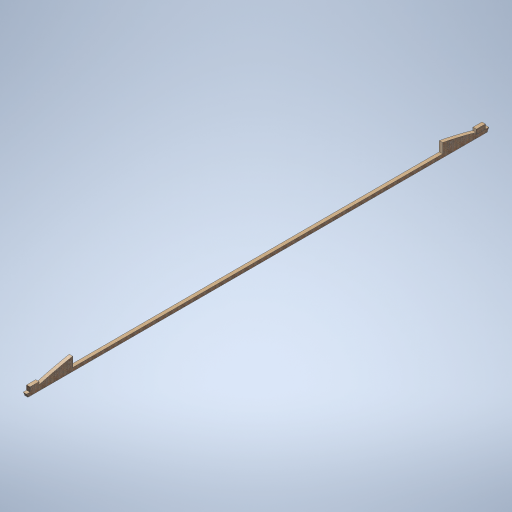
# Autodesk Inventor part: main_crossbeam
Saved by Autodesk Inventor 2024.2 (Build 282272000, 272)
## iProperties
Created: 2024-05-18
Part Number: main_crossbeam
Material: Wood Shake
Document SubType Name: Modeling
Designer: LOSTER_1
Density: 0.4 g/cm^3
Appearance: Shake - Handsplit
Author: LOSTER_1
Autodesk Inventor part; units mm, degrees
ref_plane "YZ Plane" through (0, 0, 0) normal (1, 0, 0) x (0, 1, 0)
ref_plane "XZ Plane" through (0, 0, 0) normal (0, 1, 0) x (-1, 0, 0)
ref_plane "XY Plane" through (0, 0, 0) normal (0, 0, 1) x (1, 0, 0)
sketch "Sketch1" plane through (0, 0, 0) normal (0, 0, 1) x (1, 0, 0)
  point P0 (0, 0)
sketch "Sketch2" plane through (0, 0, 0) normal (0, 0, 1) x (1, 0, 0)
  line L0 (-150, 150) -> (150, 150)
  line L1 (150, 150) -> (150, -150)
  line L2 (150, -150) -> (-150, -150)
  line L3 (-150, -150) -> (-150, 150)
  line L4 (-150, 150) -> (150, -150) construction
  line L5 (150, 150) -> (-150, -150) construction
  point P0 (0, 0)
  dimension "d0" = 300
  dimension "d1" = 300
  constraints: 12 end point, 2 midpoint, 2 parallel, 1 horizontal, 1 perpendicular
  measures "d0" distance of L1.end L2.end
  measures "d1" distance of L0.end L1.end
extrude "Extrusion1" add sketch "Sketch2" along normal mid plane 38608
sketch "Sketch4" plane through (150, 150, 19304) normal (1, 0, 0) x (0, 0, -1)
  point P0 (19304, -150)
sketch "Sketch5" plane through (-150, 150, 19304) normal (0, 1, 0) x (1, 0, 0)
  point P0 (150, 19304)
sketch "Sketch6" plane through (150, 150, 19304) normal (1, 0, 0) x (0, 0, -1)
  line L0 (38608, 0) -> (0, 0) projected
  line L1 (0, -300) -> (0, 0)
  line L2 (0, 0) -> (-1000, 0)
  line L3 (-1000, 0) -> (-875, -216.5064)
  line L4 (-875, -216.5064) -> (-695.9473, -300)
  line L5 (-695.9473, -300) -> (0, -300)
  line L6 (38608, -300) -> (38608, 0)
  line L7 (38608, 0) -> (39608, 0)
  line L8 (39608, 0) -> (39483, -216.5064)
  line L9 (39483, -216.5064) -> (39303.9473, -300)
  line L10 (39303.9473, -300) -> (38608, -300)
  point P0 (19304, -150)
  dimension "d10" = 1000
  dimension "d11" = 250
  dimension "d12" = 60
  dimension "d13" = 145
  constraints: 20 end point, 2 perpendicular, 1 parallel
  measures "d10" distance of L0.end L2.end
  measures "d11" distance of L2.end L3.end
  measures "d12" angle of L3 L2
  measures "d13" angle of L4 L3
extrude "Extrusion3" add sketch "Sketch6" against normal blind 300
sketch "Sketch7" plane through (150, 150, 20304) normal (1, 0, 0) x (0, 0, -1)
  line L0 (40303.9473, -300) -> (304.0527, -300) projected
  point P0 (20304, -150)
  constraints: 1 coincident
sketch "Sketch8" plane through (-150, 150, 20304) normal (0, 1, 0) x (1, 0, 0)
  line L0 (0, 40608) -> (0, 0) projected
  line L1 (0, 0) -> (0, 304)
  line L2 (300, 40303.9473) -> (300, 304.0527) projected
  line L3 (0, 304) -> (300, 304.0527)
  line L4 (300, 304.0527) -> (300, 1103.0527)
  line L5 (300, 1103.0527) -> (0, 1103.0527)
  line L6 (0, 1103.0527) -> (0, 304)
  line L7 (0, 40608) -> (0, 40304)
  line L8 (300, 40303.9473) -> (0, 40303.9473) projected
  line L9 (0, 40304) -> (300, 40303.9473)
  line L10 (300, 40303.9473) -> (299.8596, 39504.9473)
  line L11 (299.8596, 39504.9473) -> (0, 39504.9473)
  line L12 (0, 40303.9473) -> (0, 39504.9473)
  line L13 (0, 304.0527) -> (0, 40303.9473) projected
  point P0 (150, 20304)
  point P1 (0, 1103.0527)
  dimension "d16" = 304
  dimension "d17" = 799
  dimension "d18" = 304
  dimension "d19" = 799
  dimension "d20" = 90
  constraints: 20 end point, 5 point on line, 3 perpendicular, 1 collinear, 1 horizontal
  measures "d16" distance of L0.end L1.end
  measures "d17" distance of L2.end L4.end
  measures "d18" distance of L0.start L7.end
  measures "d19" distance of L2.start L10.end
  measures "d20" angle of L9 L10
extrude "Extrusion4" add sketch "Sketch8" along normal blind 400 contours L8 L10 L11 L0 | L2 L3 L0 L5
sketch "Sketch9" plane through (150, -150, 19999.9473) normal (1, 0, 0) x (0, 0, -1)
  line L0 (0, 0) -> (-179.0527, 83.4936) projected
  line L1 (-179.0527, 83.4936) -> (-179.0527, 0)
  line L2 (-179.0527, 0) -> (0, 0)
  line L3 (0, 0) -> (-179.0527, 83.4936)
  line L4 (0, 0) -> (39999.8946, 0) projected
  line L5 (40178.9473, 83.4936) -> (40303.9473, 300) projected
  line L6 (39999.8946, 0) -> (40178.9473, 83.4936)
  line L7 (40178.9473, 83.4936) -> (40178.9473, 0)
  line L8 (40178.9473, 0) -> (39999.8946, 0)
  point P0 (19999.9473, 150)
  constraints: 12 end point, 3 perpendicular, 1 collinear, 1 point on line, 1 vertical
extrude "Extrusion5" add sketch "Sketch9" against normal blind 300
sketch "Sketch11" plane through (150, 150, 19200.9473) normal (1, 0, 0) x (0, 0, -1)
  line L0 (39200.8946, 0) -> (0, 0) projected
  line L1 (0, 0) -> (2950, 0)
  line L2 (0, 0) -> (0, 160)
  line L3 (0, 0) -> (0, 400) projected
  line L4 (2950, 0) -> (2950, 863)
  line L5 (2950, 0) -> (3813, 0) construction
  arc A0 (2950, 863) -> (0, 160) centre (9580.862, -33503.1413) ccw
  line L6 (19200.9473, -150) -> (19200.9473, 2504.8951)
  line L7 (-799, 0) -> (38401.8946, 0)
  line L8 (38401.8946, 0) -> (38401.8946, 160)
  line L9 (35451.8946, 0) -> (35451.8946, 863)
  arc A1 (38401.8946, 160) -> (35451.8946, 863) centre (28821.0326, -33503.1413) ccw
  dimension "d25" = 2950
  dimension "d27" = 160
  dimension "d28" = 863
  dimension "d29" = 90
  dimension "d30" = 35000
  constraints: 16 end point, 6 symmetric about line, 4 point on circle, 3 perpendicular, 3 point on line, 2 centre point, 1 horizontal, 1 other
  measures "d25" distance of L0.end L1.end
  measures "d27" distance of L0.end L2.end
  measures "d28" distance of L1.end L4.end
  measures "d29" angle of L5 L4
  measures "d30" radius of A0
extrude "Extrusion6" add sketch "Sketch11" against normal blind 300
body "Solid1"
